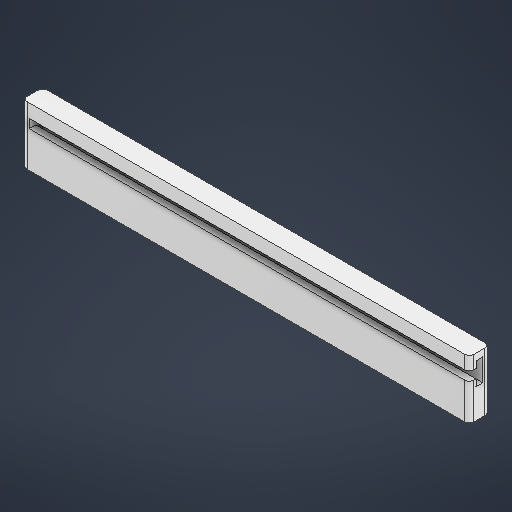
# Autodesk Inventor part: module-slot
Saved by Autodesk Inventor 2025.2 (Build 292293000, 293)
## iProperties
Created: 2025-12-31
Part Number: module-slot
Material: PC/ABS Plastic
Document SubType Name: Modeling
Designer: sam
Density: 1.1 g/cm^3
Appearance: Smooth - White
Author: sam
Autodesk Inventor part; units mm, degrees
ref_plane "YZ Plane" through (0, 0, 0) normal (1, 0, 0) x (0, 1, 0)
ref_plane "XZ Plane" through (0, 0, 0) normal (0, 1, 0) x (-1, 0, 0)
ref_plane "XY Plane" through (0, 0, 0) normal (0, 0, 1) x (1, 0, 0)
sketch "Sketch1" plane through (0, 0, 0) normal (0, 0, 1) x (1, 0, 0)
  line L0 (100, 13.1) -> (-100, 13.1)
  line L1 (-100, 13.1) -> (-100, -13.1)
  line L2 (-100, -13.1) -> (100, -13.1)
  line L3 (100, -13.1) -> (100, 13.1)
  line L4 (100, 13.1) -> (-100, -13.1) construction
  line L5 (-100, 13.1) -> (100, -13.1) construction
  point P0 (0, 0)
  dimension "d0" = 200
  dimension "d1" = 26.2
  constraints: 12 end point, 2 midpoint, 2 parallel, 1 horizontal, 1 perpendicular
  measures "d0" distance of L2.end L1.end
  measures "d1" distance of L1.end L0.end
extrude "Extrusion1" add sketch "Sketch1" along normal blind 9
sketch "Sketch2" plane through (100, -13.1, 0) normal (1, 0, 0) x (0, 0, -1)
  line L0 (0, 0) -> (0, 26.2) projected
  line L1 (0, 26.2) -> (-9, 26.2) projected
  line L2 (-9, 0) -> (-9, 26.2) projected
  line L3 (0, 0) -> (-9, 0) projected
  line L4 (-9, 26.2) -> (-9, 0) projected
  line L5 (-9, 26.2) -> (-3, 26.2)
  line L6 (-3, 26.2) -> (-3, 23.2)
  line L7 (-3, 23.2) -> (-9, 23.2)
  line L8 (-9, 23.2) -> (-9, 26.2)
  line L9 (-9, 23.2) -> (-6, 23.2)
  line L10 (-6, 23.2) -> (-6, 20.2)
  line L11 (-6, 20.2) -> (-9, 20.2)
  line L12 (-9, 20.2) -> (-9, 23.2)
  line L13 (-9, 26.2) -> (-3, 26.2)
  line L14 (-3, 26.2) -> (-3, 10.2)
  line L15 (-3, 10.2) -> (-9, 10.2)
  line L16 (-9, 10.2) -> (-9, 26.2)
  line L17 (-9, 10.2) -> (-3, 10.2)
  line L18 (-3, 10.2) -> (-3, 13.2)
  line L19 (-3, 13.2) -> (-9, 13.2)
  line L20 (-9, 13.2) -> (-9, 10.2)
  line L21 (-9, 13.2) -> (-6, 13.2)
  line L22 (-6, 13.2) -> (-6, 16.2)
  line L23 (-6, 16.2) -> (-9, 16.2)
  line L24 (-9, 16.2) -> (-9, 13.2)
  point P0 (0, 13.1)
  point P1 (-3, 23.2)
  point P2 (-9, 20.2)
  dimension "d4" = 6
  dimension "d5" = 3
  dimension "d6" = 3
  dimension "d7" = 3
  dimension "d8" = 16
  dimension "d9" = 3
  dimension "d10" = 3
  dimension "d11" = 3
  constraints: 40 end point, 10 parallel, 5 horizontal, 5 perpendicular, 1 point on line
  measures "d4" distance of L6.end L7.end
  measures "d5" distance of L5.end L6.end
  measures "d6" distance of L10.end L11.end
  measures "d7" distance of L9.end L10.end
  measures "d8" distance of L13.end L14.end
  measures "d9" distance of L18.end L17.end
  measures "d10" distance of L23.end L22.end
  measures "d11" distance of L22.end L21.end
extrude "Extrusion2" cut sketch "Sketch2" against normal blind 197 contours L14 L19 L22 L23 L2 L11 L10 L7
fillet "Fillet1" radius 2 5 edges at (100, 10.1, 9) (100, -5, 9) (-100, 0, 9) (100, 0, 0) (-100, 0, 0)
body "Solid1"
